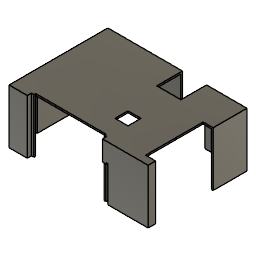
Case (Autodesk Fusion 360 design; units mm, degrees)
Autodesk Fusion 360 part; units mm, degrees
ref_plane "Arbeitsebene1" through (-71.75, -25.15, 142.25) normal (0, 0, 1) x (0, -1, 0)
sketch "Skizze1" plane through (0, 0, 142.25) normal (0, 0, 1) x (1, 0, 0)
  line L0 (-35.7, -26.35) -> (-35.7, -31.2)
  line L1 (-35.7, -26.35) -> (-40.5, -26.35)
  line L2 (-40.5, -26.35) -> (-40.5, -28.35)
  line L3 (-35.5, -1) -> (-35.5, -31)
  line L4 (-33.5, -26.15) -> (-40.5, -26.15)
  line L5 (-40.5, -28.35) -> (-37.7, -28.35)
  line L6 (-37.7, -28.35) -> (-37.7, -33.2)
  line L7 (-37.7, -33.2) -> (15.7, -33.2)
  line L8 (-35.7, -31.2) -> (13.7, -31.2)
  line L9 (15.7, -33.2) -> (15.7, 82.2)
  line L10 (-127.3, -26.35) -> (-127.3, -31.2)
  line L11 (-127.3, -26.35) -> (-122.5, -26.35)
  line L12 (-103, -26.15) -> (-129.5, -26.15)
  line L13 (-127.5, -1) -> (-127.5, -31)
  line L14 (-122.5, -26.35) -> (-122.5, -28.35)
  line L15 (-122.5, -28.35) -> (-125.3, -28.35)
  line L16 (-125.3, -28.35) -> (-125.3, -33.2)
  line L17 (-125.3, -33.2) -> (-146.7, -33.2)
  line L18 (-127.3, -31.2) -> (-144.7, -31.2)
  line L19 (-144.7, -31.2) -> (-144.7, 80.2)
  line L20 (-146.7, -33.2) -> (-146.7, 82.2)
  line L21 (15.7, 82.2) -> (-146.7, 82.2)
  line L22 (-144.7, 80.2) -> (13.7, 80.2)
  line L23 (13.7, -31.2) -> (13.7, 80.2)
  line L24 (-122.5, -26.35) -> (-40.5, -26.35)
  dimension "d51" = 0.2
  dimension "d52" = 0.2
  dimension "d53" = 4.8
  dimension "d54" = 2
  dimension "d55" = 4.85
  dimension "d56" = 2.8
  dimension "d57" = 4.85
  dimension "d58" = 53.4
  dimension "d59" = 49.4
  dimension "d60" = 115.4
  dimension "d61" = 0.2
  dimension "d62" = 0.2
  dimension "d63" = 4.8
  dimension "d64" = 4.85
  dimension "d65" = 2
  dimension "d66" = 2.8
  dimension "d67" = 4.85
  dimension "d68" = 21.4
  dimension "d69" = 17.4
  dimension "d70" = 111.4
  dimension "d71" = 115.4
  dimension "d72" = 158.4
  dimension "d73" = 162.4
  dimension "d74" = 111.4
  constraint vertical L0
  constraint perpendicular L0 L1
  constraint perpendicular L1 L2
  constraint perpendicular L2 L5
  constraint perpendicular L5 L6
  constraint perpendicular L6 L7
  constraint perpendicular L3 L8
  constraint perpendicular L7 L9
  constraint vertical L10
  constraint perpendicular L10 L11
  constraint perpendicular L11 L14
  constraint perpendicular L14 L15
  constraint perpendicular L15 L16
  constraint perpendicular L16 L17
  constraint perpendicular L10 L18
  constraint perpendicular L17 L20
  constraint perpendicular L19 L22
  constraint perpendicular L8 L23
  measures "d51" distance of L0 L3
  measures "d52" distance of L1 L4
  measures "d53" distance of L0.start L1.end
  measures "d54" distance of L1.end L2.end
  measures "d55" distance of L0.start L0.end
  measures "d56" distance of L2.end L5.end
  measures "d57" distance of L5.end L6.end
  measures "d58" distance of L6.end L7.end
  measures "d59" distance of L0.end L8.end
  measures "d60" distance of L7.end L9.end
  measures "d61" distance of L11 L12
  measures "d62" distance of L10 L13
  measures "d63" distance of L10.start L11.end
  measures "d64" distance of L10.start L10.end
  measures "d65" distance of L11.end L14.end
  measures "d66" distance of L14.end L15.end
  measures "d67" distance of L15.end L16.end
  measures "d68" distance of L16.end L17.end
  measures "d69" distance of L10.end L18.end
  measures "d70" distance of L18.end L19.end
  measures "d71" distance of L17.end L20.end
  measures "d72" distance of L19.end L22.end
  measures "d73" distance of L9.end L20.end
  measures "d74" distance of L8.end L22.end
extrude "Extrusion1" add sketch "Skizze1" along normal blind 2
extrude "Extrusion2" add sketch "Skizze1" against normal blind 61.5 contours L0 L1 L2 L5 L6 L7 L8 L9 L10 L11 L14 L15 L16 L17 L18 L19 L20 L21 L22 L23
box "Grundkörper Quader5" cut length 67 width 11.65 height -63.5 placed x (0, 1, 0) y (1, 0, 0) z (0, 0, -1) at (4.05, -24.3544, 80.75)
box "Grundkörper Quader1" cut length 40 width 2 height -41.5 placed x (0, -1, 0) y (-1, 0, 0) z (0, 0, -1) at (-31.3, 6.7996, 80.75)
box "Grundkörper Quader2" cut length 2 width 4.4 height -40 placed x (0, 1, 0) y (1, 0, 0) z (0, 0, -1) at (-37.7, -33.2, 80.75)
sketch "Skizze10" plane through (0, 82.2, 0) normal (0, 1, 0) x (-1, 0, 0)
  line L0 (146.7, 80.75) -> (146.7, 144.25)
  line L1 (146.7, 144.25) -> (-15.7, 144.25)
  line L2 (-15.7, 144.25) -> (-15.7, 80.75)
  line L3 (-15.7, 80.75) -> (146.7, 80.75)
  line L4 (146.7, 80.75) -> (124.7, 80.75) construction
  line L5 (124.7, 80.75) -> (124.7, 92.75) construction
  line L6 (124.7, 92.75) -> (146.7, 92.75) construction
  line L7 (146.7, 92.75) -> (146.7, 80.75) construction
  line L8 (146.7, 80.75) -> (140.7, 80.75) construction
  line L9 (140.7, 80.75) -> (140.7, 86.75) construction
  line L10 (140.7, 86.75) -> (146.7, 86.75) construction
  line L11 (146.7, 86.75) -> (146.7, 80.75) construction
  line L12 (140.7, 86.75) -> (124.7, 86.75)
  line L13 (124.7, 86.75) -> (124.7, 92.75)
  line L14 (124.7, 92.75) -> (140.7, 92.75)
  line L15 (140.7, 92.75) -> (140.7, 86.75)
  line L16 (58.5044, 80.75) -> (88.5044, 80.75) construction
  line L17 (88.5044, 80.75) -> (88.5044, 92.75) construction
  line L18 (88.5044, 92.75) -> (58.5044, 92.75) construction
  line L19 (58.5044, 92.75) -> (58.5044, 80.75) construction
  line L20 (58.5044, 80.75) -> (63.5044, 80.75) construction
  line L21 (63.5044, 80.75) -> (63.5044, 85.75) construction
  line L22 (63.5044, 85.75) -> (58.5044, 85.75) construction
  line L23 (58.5044, 85.75) -> (58.5044, 80.75) construction
  line L24 (63.5044, 85.75) -> (88.5044, 85.75)
  line L25 (88.5044, 85.75) -> (88.5044, 92.75)
  line L26 (88.5044, 92.75) -> (63.5044, 92.75)
  line L27 (63.5044, 92.75) -> (63.5044, 85.75)
  dimension "d87" = 22
  dimension "d88" = 12
  dimension "d89" = 6
  dimension "d90" = 6
  dimension "d93" = 30
  dimension "d94" = 12
  dimension "d95" = 5
  dimension "d96" = 5
  constraint horizontal L4
  constraint vertical L5
  constraint horizontal L6
  constraint vertical L7
  constraint coincident L0.start L3.end
  constraint horizontal L8
  constraint vertical L9
  constraint horizontal L10
  constraint vertical L11
  constraint horizontal L12
  constraint vertical L13
  constraint horizontal L14
  constraint vertical L15
  constraint horizontal L16
  constraint vertical L17
  constraint horizontal L18
  constraint vertical L19
  constraint coincident L3 L16.start
  constraint horizontal L20
  constraint vertical L21
  constraint horizontal L22
  constraint vertical L23
  constraint horizontal L24
  constraint vertical L25
  constraint horizontal L26
  constraint vertical L27
  measures "d87" distance of L0.start L4.end
  measures "d88" distance of L0.start L6.end
  measures "d89" distance of L0.start L8.end
  measures "d90" distance of L0.start L10.end
  measures "d93" distance of L16.start L16.end
  measures "d94" distance of L16.start L18.end
  measures "d95" distance of L16.start L20.end
  measures "d96" distance of L16.start L22.end
extrude "Extrusion3" cut sketch "Skizze10" against normal blind 2 contours L12 L13 L14 L15 | L24 L25 L26 L27
box "Grundkörper Quader3" cut length 30 width 28 height -63.5 placed x (0, 1, 0) y (1, 0, 0) z (0, 0, -1) at (-59.529, 52.2, 80.75)
box "Grundkörper Quader4" cut length 15 width 15 height -2 placed x (0, -1, 0) y (1, 0, 0) z (0, 0, 1) at (-51, 10, 144.25)
sketch "Skizze14" plane through (-146.7, 0, 0) normal (-1, 0, 0) x (0, -1, 0)
  line L0 (33.2, 80.75) -> (33.2, 144.25)
  line L1 (33.2, 144.25) -> (-82.2, 144.25)
  line L2 (-82.2, 144.25) -> (-82.2, 80.75)
  line L3 (-82.2, 80.75) -> (33.2, 80.75)
  line L4 (33.2, 80.75) -> (21.2, 80.75) construction
  line L5 (33.2, 80.75) -> (2.2, 80.75) construction
  line L6 (2.2, 80.75) -> (2.2, 137.75) construction
  line L7 (2.2, 137.75) -> (33.2, 137.75) construction
  line L8 (33.2, 137.75) -> (33.2, 80.75) construction
  line L9 (21.2, 80.75) -> (2.2, 80.75)
  line L10 (2.2, 80.75) -> (2.2, 137.75)
  line L11 (2.2, 137.75) -> (21.2, 137.75)
  line L12 (21.2, 137.75) -> (21.2, 80.75)
  dimension "d112" = 12
  dimension "d114" = 31
  dimension "d115" = 57
  constraint horizontal L4
  constraint coincident L0.start L3.end
  constraint horizontal L5
  constraint vertical L6
  constraint horizontal L7
  constraint vertical L8
  constraint horizontal L9
  constraint vertical L10
  constraint horizontal L11
  constraint vertical L12
  measures "d112" distance of L0.start L4.end
  measures "d114" distance of L0.start L5.end
  measures "d115" distance of L0.start L7.end
extrude "Extrusion4" cut sketch "Skizze14" against normal blind 2 contours L3 L9 L10 L11 L12
